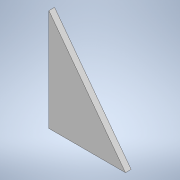
# Autodesk Inventor part: Maze part 4
Saved by Autodesk Inventor 2021 (Build 250183000, 183)
## iProperties
Created: 2021-06-18
Part Number: Maze part 4
Material: Generic
Document SubType Name: Modeling
Designer: Dell
Density: 1 g/cm^3
Appearance: Default
Author: Dell
Autodesk Inventor part; units mm, degrees
ref_plane "YZ Plane" through (0, 0, 0) normal (1, 0, 0) x (0, 1, 0)
ref_plane "XZ Plane" through (0, 0, 0) normal (0, 1, 0) x (-1, 0, 0)
ref_plane "XY Plane" through (0, 0, 0) normal (0, 0, 1) x (1, 0, 0)
sketch "Sketch1" plane through (0, 0, 0) normal (0, 0, 1) x (1, 0, 0)
  line L0 (-4.3248, 10.2004) -> (-4.3248, -7.7977)
  line L1 (-4.3248, -7.7977) -> (9.1738, -7.7977)
  line L2 (9.1738, -7.7977) -> (-4.3248, 10.2004)
  point P0 (0, 0)
  constraints: 6 end point, 1 perpendicular, 1 vertical
extrude "Extrusion1" add sketch "Sketch1" along normal blind 1
body "Solid1"
